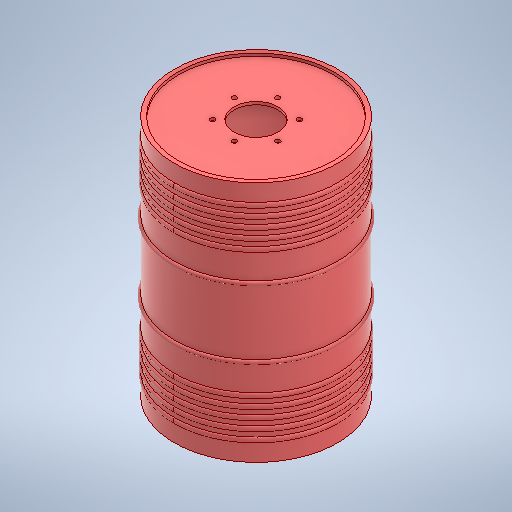
# Autodesk Inventor part: drum oil
Saved by Autodesk Inventor 2025.2 (Build 292293000, 293)
## iProperties
Created: 2021-05-10
Part Number: drum oil
Material: Generic
Document SubType Name: Modeling
Designer: Gold D.Roger
Density: 1 g/cm^3
Appearance: Smooth - Red
Author: Gold D.Roger
Autodesk Inventor part; units mm, degrees
ref_plane "YZ Plane" through (0, 0, 0) normal (1, 0, 0) x (0, 1, 0)
ref_plane "XZ Plane" through (0, 0, 0) normal (0, 1, 0) x (-1, 0, 0)
ref_plane "XY Plane" through (0, 0, 0) normal (0, 0, 1) x (1, 0, 0)
sketch "Sketch1" plane through (0, 0, 0) normal (0, 1, 0) x (-1, 0, 0)
  circle A0 centre (0, 0) radius 290
  dimension "d0" = 580
  constraints: 1 centre point, 1 coincident
  measures "d0" diameter of A0
extrude "Extrusion1" add sketch "Sketch1" along normal blind 860
shell "Shell1" thickness 15 removed faces 1 at (10.7292, 860, -77.9435)
sketch "Sketch2" plane through (0, 0, 0) normal (1, 0, 0) x (0, 1, 0)
  line L0 (0, 290) -> (860, 290) projected
  line L1 (430, 290) -> (430, -229.4954)
  circle A0 centre (551.2756, 290) radius 7.5
  ellipse E0 centre (655.1144, 288.0629) end of major axis (655.1144, 282.2424) minor radius 9.6727
  ellipse E1 centre (689.1144, 288.0629) end of major axis (689.1144, 282.2424) minor radius 9.6727
  ellipse E2 centre (723.1144, 288.0629) end of major axis (723.1144, 282.2424) minor radius 9.6727
  ellipse E3 centre (757.1144, 288.0629) end of major axis (757.1144, 282.2424) minor radius 9.6727
  ellipse E4 centre (791.1144, 288.0629) end of major axis (791.1144, 282.2424) minor radius 9.6727
  line L2 (829.0253, 0) -> (621.6232, 0)
  point P0 (0, 0)
  point P1 (558.7756, 290)
  point P2 (543.7756, 290)
  dimension "d4" = 15
  dimension "d7" = 34
  constraints: 6 centre point, 4 end point, 2 horizontal, 1 midpoint, 1 point on line, 1 vertical, 9 other
  measures "d4" diameter of A0
  measures "d7" distance of E0.centre E1.centre
revolve "Revolution1" add sketch "Sketch2" angle 360 about axis through (0, 829.0253, 0) along (0, -1, 0) picked at (551.5769, 292.4818) contours A0 L0 | E0 L0 | L0 E0 | E1 L0 | L0 E1 | E2 L0 | L0 E2 | E3 L0 | L0 E3 | E4 L0 | L0 E4
ref_plane "Work Plane1" through (0, 430, 0) normal (0, 1, 0) x (1, 0, 0)
mirror "Mirror1" about plane through (0, 430, 0) normal (0, 1, 0) of "Revolution1"
ref_plane "Work Plane2" through (0, 850, 0) normal (0, 1, 0) x (1, 0, 0)
sketch "Sketch3" plane through (0, 850, 0) normal (0, 1, 0) x (1, 0, 0)
  circle A0 centre (0, 0) radius 275 projected
extrude "Extrusion2" add sketch "Sketch3" against normal blind 10
scale "Scale1" factors (0.5, 0.5, 0.5) then translate (0, 213.75, 0) bodies 1
sketch "Sketch6" plane through (0, 638.75, 0) normal (0, 1, 0) x (1, 0, 0)
  arc A0 (-39.2176, 0) -> (39.2176, 0) centre (0, 0) ccw
  line L0 (-39.2176, 0) -> (-66.04, 0)
  arc A1 (-66.04, 0) -> (66.04, 0) centre (0, 0) ccw
  line L1 (39.2176, 0) -> (66.04, 0)
  circle A2 centre (-38.5792, -38.5792) radius 4.3434
  circle A3 centre (52.7001, -14.121) radius 4.3434
  arc A4 (16.2927, -48.9386) -> (11.9493, -56.4616) centre (14.121, -52.7001) ccw
  arc A5 (11.9493, -56.4616) -> (16.2927, -48.9386) centre (14.121, -52.7001) ccw
  line L2 (39.2176, 0) -> (66.04, 0)
  arc A6 (66.04, 0) -> (-66.04, 0) centre (0, 0) ccw
  line L3 (-39.2176, 0) -> (-66.04, 0)
  arc A7 (39.2176, 0) -> (-39.2176, 0) centre (0, 0) ccw
  circle A8 centre (-52.7001, 14.121) radius 4.3434
  arc A9 (-16.2927, 48.9386) -> (-11.9493, 56.4616) centre (-14.121, 52.7001) ccw
  arc A10 (-11.9493, 56.4616) -> (-16.2927, 48.9386) centre (-14.121, 52.7001) ccw
  circle A11 centre (38.5792, 38.5792) radius 4.3434
  point P0 (0, 0)
  constraints: 16 point on circle, 12 centre point, 8 end point
extrude "Extrusion5" cut sketch "Sketch6" against normal blind 5 contours A2 | A3 | A5 A4 | A8 | A10 A9 | A11
extrude "Extrusion6" cut sketch "Sketch6" against normal blind 5 contours A7 A0
body "Solid1"
